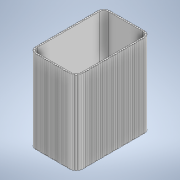
# Autodesk Inventor part: CircleContainer
Saved by Autodesk Inventor 2020 (Build 240168000, 168)
## iProperties
Created: 2024-02-26
Part Number: CircleContainer
Material: Generic
Document SubType Name: Modeling
Designer: smz3rm
Density: 1 g/cm^3
Appearance: Default
Author: smz3rm
Autodesk Inventor part; units mm, degrees
ref_plane "YZ Plane" through (0, 0, 0) normal (1, 0, 0) x (0, 1, 0)
ref_plane "XZ Plane" through (0, 0, 0) normal (0, 1, 0) x (-1, 0, 0)
ref_plane "XY Plane" through (0, 0, 0) normal (0, 0, 1) x (1, 0, 0)
sketch "Sketch3" plane through (0, 0, 0) normal (0, 1, 0) x (-1, 0, 0)
  line L0 (-31.4159, 66.9414) -> (31.4159, 66.9414)
  line L1 (41.4159, 56.9414) -> (41.4159, -56.9414)
  line L2 (31.4159, -66.9414) -> (-31.4159, -66.9414)
  line L3 (-41.4159, -56.9414) -> (-41.4159, 56.9414)
  line L4 (-41.4159, 66.9414) -> (41.4159, -66.9414) construction
  line L5 (41.4159, 66.9414) -> (-41.4159, -66.9414) construction
  arc A0 (41.4159, 56.9414) -> (31.4159, 66.9414) centre (31.4159, 56.9414) ccw
  arc A1 (-31.4159, 66.9414) -> (-41.4159, 56.9414) centre (-31.4159, 56.9414) ccw
  arc A2 (31.4159, -66.9414) -> (41.4159, -56.9414) centre (31.4159, -56.9414) ccw
  arc A3 (-41.4159, -56.9414) -> (-31.4159, -66.9414) centre (-31.4159, -56.9414) ccw
  line L6 (60.8818, 0) -> (-60.8818, 0) projected
  line L7 (0, -96.6174) -> (0, 96.6174) projected
  circle A4 centre (31.4159, 66.9414) radius 1.9635
  circle A5 centre (35.2428, 66.1802) radius 1.9635
  circle A6 centre (38.487, 64.0124) radius 1.9635
  circle A7 centre (40.6547, 60.7682) radius 1.9635
  circle A8 centre (41.4159, 56.9414) radius 1.9635
  circle A9 centre (41.4159, 53.0144) radius 1.9635
  circle A10 centre (41.4159, 49.0874) radius 1.9635
  circle A11 centre (41.4159, 45.1604) radius 1.9635
  circle A12 centre (41.4159, 41.2334) radius 1.9635
  circle A13 centre (41.4159, 37.3064) radius 1.9635
  circle A14 centre (41.4159, 33.3794) radius 1.9635
  circle A15 centre (41.4159, 29.4524) radius 1.9635
  circle A16 centre (41.4159, 25.5254) radius 1.9635
  circle A17 centre (41.4159, 21.5984) radius 1.9635
  circle A18 centre (41.4159, 17.6715) radius 1.9635
  circle A19 centre (41.4159, 13.7445) radius 1.9635
  circle A20 centre (41.4159, 9.8175) radius 1.9635
  circle A21 centre (41.4159, 5.8905) radius 1.9635
  circle A22 centre (41.4159, 1.9635) radius 1.9635
  circle A23 centre (41.4159, -1.9635) radius 1.9635
  circle A24 centre (41.4159, -5.8905) radius 1.9635
  circle A25 centre (41.4159, -9.8175) radius 1.9635
  circle A26 centre (41.4159, -13.7445) radius 1.9635
  circle A27 centre (41.4159, -17.6715) radius 1.9635
  circle A28 centre (41.4159, -21.5984) radius 1.9635
  circle A29 centre (41.4159, -25.5254) radius 1.9635
  circle A30 centre (41.4159, -29.4524) radius 1.9635
  circle A31 centre (41.4159, -33.3794) radius 1.9635
  circle A32 centre (41.4159, -37.3064) radius 1.9635
  circle A33 centre (41.4159, -41.2334) radius 1.9635
  circle A34 centre (41.4159, -45.1604) radius 1.9635
  circle A35 centre (41.4159, -49.0874) radius 1.9635
  circle A36 centre (41.4159, -53.0144) radius 1.9635
  circle A37 centre (-41.4159, 56.9414) radius 1.9635
  circle A38 centre (-41.4159, 53.0144) radius 1.9635
  circle A39 centre (-41.4159, 49.0874) radius 1.9635
  circle A40 centre (-41.4159, 45.1604) radius 1.9635
  circle A41 centre (-41.4159, 41.2334) radius 1.9635
  circle A42 centre (-41.4159, 37.3064) radius 1.9635
  circle A43 centre (-41.4159, 33.3794) radius 1.9635
  circle A44 centre (-41.4159, 29.4524) radius 1.9635
  circle A45 centre (-41.4159, 25.5254) radius 1.9635
  circle A46 centre (-41.4159, 21.5984) radius 1.9635
  circle A47 centre (-41.4159, 17.6715) radius 1.9635
  circle A48 centre (-41.4159, 13.7445) radius 1.9635
  circle A49 centre (-41.4159, 9.8175) radius 1.9635
  circle A50 centre (-41.4159, 5.8905) radius 1.9635
  circle A51 centre (-41.4159, 1.9635) radius 1.9635
  circle A52 centre (-41.4159, -1.9635) radius 1.9635
  circle A53 centre (-41.4159, -5.8905) radius 1.9635
  circle A54 centre (-41.4159, -9.8175) radius 1.9635
  circle A55 centre (-41.4159, -13.7445) radius 1.9635
  circle A56 centre (-41.4159, -17.6715) radius 1.9635
  circle A57 centre (-41.4159, -21.5984) radius 1.9635
  circle A58 centre (-41.4159, -25.5254) radius 1.9635
  circle A59 centre (-41.4159, -29.4524) radius 1.9635
  circle A60 centre (-41.4159, -33.3794) radius 1.9635
  circle A61 centre (-41.4159, -37.3064) radius 1.9635
  circle A62 centre (-41.4159, -41.2334) radius 1.9635
  circle A63 centre (-41.4159, -45.1604) radius 1.9635
  circle A64 centre (-41.4159, -49.0874) radius 1.9635
  circle A65 centre (-41.4159, -53.0144) radius 1.9635
  circle A66 centre (31.4159, -66.9414) radius 1.9635
  circle A67 centre (35.2428, -66.1802) radius 1.9635
  circle A68 centre (38.487, -64.0124) radius 1.9635
  circle A69 centre (40.6547, -60.7682) radius 1.9635
  circle A70 centre (41.4159, -56.9414) radius 1.9635
  circle A71 centre (-31.4159, 66.9414) radius 1.9635
  circle A72 centre (-35.2428, 66.1802) radius 1.9635
  circle A73 centre (-38.487, 64.0124) radius 1.9635
  circle A74 centre (-40.6547, 60.7682) radius 1.9635
  circle A75 centre (-41.4159, 56.9414) radius 1.9635
  circle A76 centre (-31.4159, -66.9414) radius 1.9635
  circle A77 centre (-35.2428, -66.1802) radius 1.9635
  circle A78 centre (-38.487, -64.0124) radius 1.9635
  circle A79 centre (-40.6547, -60.7682) radius 1.9635
  circle A80 centre (31.4159, -66.9414) radius 1.9635
  circle A81 centre (27.4889, 66.9414) radius 1.9635
  circle A82 centre (27.4889, -66.9414) radius 1.9635
  circle A83 centre (23.5619, 66.9414) radius 1.9635
  circle A84 centre (23.5619, -66.9414) radius 1.9635
  circle A85 centre (19.635, 66.9414) radius 1.9635
  circle A86 centre (19.635, -66.9414) radius 1.9635
  circle A87 centre (15.708, 66.9414) radius 1.9635
  circle A88 centre (15.708, -66.9414) radius 1.9635
  circle A89 centre (11.781, 66.9414) radius 1.9635
  circle A90 centre (11.781, -66.9414) radius 1.9635
  circle A91 centre (7.854, 66.9414) radius 1.9635
  circle A92 centre (7.854, -66.9414) radius 1.9635
  circle A93 centre (3.927, 66.9414) radius 1.9635
  circle A94 centre (3.927, -66.9414) radius 1.9635
  circle A95 centre (0, 66.9414) radius 1.9635
  circle A96 centre (0, -66.9414) radius 1.9635
  circle A97 centre (-3.927, 66.9414) radius 1.9635
  circle A98 centre (-3.927, -66.9414) radius 1.9635
  circle A99 centre (-7.854, 66.9414) radius 1.9635
  circle A100 centre (-7.854, -66.9414) radius 1.9635
  circle A101 centre (-11.781, 66.9414) radius 1.9635
  circle A102 centre (-11.781, -66.9414) radius 1.9635
  circle A103 centre (-15.708, 66.9414) radius 1.9635
  circle A104 centre (-15.708, -66.9414) radius 1.9635
  circle A105 centre (-19.635, 66.9414) radius 1.9635
  circle A106 centre (-19.635, -66.9414) radius 1.9635
  circle A107 centre (-23.5619, 66.9414) radius 1.9635
  circle A108 centre (-23.5619, -66.9414) radius 1.9635
  circle A109 centre (-27.4889, 66.9414) radius 1.9635
  circle A110 centre (-27.4889, -66.9414) radius 1.9635
  circle A111 centre (-41.4159, -56.9414) radius 1.9635
  point P0 (0, 0)
  point P1 (33.3727, 66.7785)
  point P2 (29.4524, 66.9414)
  point P3 (25.5254, 66.9414)
  point P4 (21.5984, 66.9414)
  point P5 (17.6715, 66.9414)
  point P6 (13.7445, 66.9414)
  point P7 (9.8175, 66.9414)
  point P8 (5.8905, 66.9414)
  point P9 (1.9635, 66.9414)
  point P10 (-1.9635, 66.9414)
  point P11 (-5.8905, 66.9414)
  point P12 (-9.8175, 66.9414)
  point P13 (-13.7445, 66.9414)
  point P14 (-17.6715, 66.9414)
  point P15 (-21.5984, 66.9414)
  point P16 (-25.5254, 66.9414)
  point P17 (-29.4524, 66.9414)
  point P18 (-33.3727, 66.7785)
  point P19 (-36.9882, 65.2809)
  point P20 (-39.7555, 62.5137)
  point P21 (-41.2531, 58.8981)
  point P22 (-41.4159, 54.9779)
  point P23 (-41.4159, 51.0509)
  point P24 (-41.4159, 47.1239)
  point P25 (-41.4159, 43.1969)
  point P26 (-41.4159, 39.2699)
  point P27 (-41.4159, 35.3429)
  point P28 (-41.4159, 31.4159)
  point P29 (-41.4159, 27.4889)
  point P30 (-41.4159, 23.5619)
  point P31 (-41.4159, 19.635)
  point P32 (-41.4159, 15.708)
  point P33 (-41.4159, 11.781)
  point P34 (-41.4159, 7.854)
  point P35 (-41.4159, 3.927)
  point P36 (-41.4159, 0)
  point P37 (-41.4159, -3.927)
  point P38 (-41.4159, -7.854)
  point P39 (-41.4159, -11.781)
  point P40 (-41.4159, -15.708)
  point P41 (-41.4159, -19.635)
  point P42 (-41.4159, -23.5619)
  point P43 (-41.4159, -27.4889)
  point P44 (-41.4159, -31.4159)
  point P45 (-41.4159, -35.3429)
  point P46 (-41.4159, -39.2699)
  point P47 (-41.4159, -43.1969)
  point P48 (-41.4159, -47.1239)
  point P49 (-41.4159, -51.0509)
  point P50 (-41.4159, -54.9779)
  point P51 (-41.2531, -58.8981)
  point P52 (-39.7555, -62.5137)
  point P53 (-36.9882, -65.2809)
  point P54 (-33.3727, -66.7785)
  point P55 (-29.4524, -66.9414)
  point P56 (-25.5254, -66.9414)
  point P57 (-21.5984, -66.9414)
  point P58 (-17.6715, -66.9414)
  point P59 (-13.7445, -66.9414)
  point P60 (-9.8175, -66.9414)
  point P61 (-5.8905, -66.9414)
  point P62 (-1.9635, -66.9414)
  point P63 (1.9635, -66.9414)
  point P64 (5.8905, -66.9414)
  point P65 (9.8175, -66.9414)
  point P66 (13.7445, -66.9414)
  point P67 (17.6715, -66.9414)
  point P68 (21.5984, -66.9414)
  point P69 (25.5254, -66.9414)
  point P70 (29.4524, -66.9414)
  point P71 (33.3727, -66.7785)
  point P72 (36.9882, -65.2809)
  point P73 (39.7555, -62.5137)
  point P74 (41.2531, -58.8981)
  point P75 (41.4159, -54.9779)
  point P76 (41.4159, -51.0509)
  point P77 (41.4159, -47.1239)
  point P78 (41.4159, -43.1969)
  point P79 (41.4159, -39.2699)
  point P80 (41.4159, -35.3429)
  point P81 (41.4159, -31.4159)
  point P82 (41.4159, -27.4889)
  point P83 (41.4159, -23.5619)
  point P84 (41.4159, -19.635)
  point P85 (41.4159, -15.708)
  point P86 (41.4159, -11.781)
  point P87 (41.4159, -7.854)
  point P88 (41.4159, -3.927)
  point P89 (41.4159, 0)
  point P90 (41.4159, 3.927)
  point P91 (41.4159, 7.854)
  point P92 (41.4159, 11.781)
  point P93 (41.4159, 15.708)
  point P94 (41.4159, 19.635)
  point P95 (41.4159, 23.5619)
  point P96 (41.4159, 27.4889)
  point P97 (41.4159, 31.4159)
  point P98 (41.4159, 35.3429)
  point P99 (41.4159, 39.2699)
  point P100 (41.4159, 43.1969)
  point P101 (41.4159, 47.1239)
  point P102 (41.4159, 51.0509)
  point P103 (41.4159, 54.9779)
  point P104 (41.2531, 58.8981)
  point P105 (39.7555, 62.5137)
  point P106 (36.9882, 65.2809)
  dimension "d50" = 10
  dimension "d51" = 10
  dimension "d52" = 10
  dimension "d53" = 10
  dimension "d66" = 113.8827
  dimension "d67" = 62.8319
  dimension "d68" = 3.927
  dimension "d71" = 90
  dimension "d75" = 3.927
  dimension "d78" = 82.8319
  dimension "d83" = 133.8827
  dimension "d86" = 3.927
  constraints: 112 centre point, 15 symmetric about line, 12 end point, 8 point on circle, 8 point on line, 8 tangent, 3 horizontal, 2 midpoint, 2 parallel, 2 vertical, 1 coincident, 1 perpendicular, 200 other
  measures "d50" radius of A0
  measures "d51" radius of A1
  measures "d52" radius of A2
  measures "d53" radius of A3
  measures "d66" distance of L1.end L1.start
  measures "d67" distance of L2.end L2.start
  measures "d68" diameter of A4
  measures "d75" distance of A8.centre A9.centre
  measures "d78" distance of A8.centre A37.centre
  measures "d83" distance of A4.centre A80.centre
  measures "d86" distance of A4.centre A81.centre
extrude "Extrusion3" add sketch "Sketch3" along normal blind 152.4
sketch "Sketch4" plane through (0, 152.4, 0) normal (0, 1, 0) x (1, 0, 0)
  arc A0 (-41.4159, -56.9414) -> (-31.4159, -66.9414) centre (-31.4159, -56.9414) ccw
  arc A1 (-31.4159, 66.9414) -> (-41.4159, 56.9414) centre (-31.4159, 56.9414) ccw
  arc A2 (31.4159, -66.9414) -> (41.4159, -56.9414) centre (31.4159, -56.9414) ccw
  arc A3 (41.4159, 56.9414) -> (31.4159, 66.9414) centre (31.4159, 56.9414) ccw
  line L0 (-41.4159, -56.9414) -> (-41.4159, 56.9414)
  line L1 (-31.4159, -66.9414) -> (31.4159, -66.9414)
  line L2 (41.4159, -56.9414) -> (41.4159, 56.9414)
  line L3 (-31.4159, 66.9414) -> (31.4159, 66.9414)
  line L4 (-60.8818, 0) -> (60.8818, 0) projected
  line L5 (0, 96.6174) -> (0, -96.6174) projected
  line L6 (-40.2159, 56.9414) -> (-40.2159, -56.9414)
  arc A4 (-40.2159, -56.9414) -> (-31.4159, -65.7414) centre (-31.4159, -56.9414) ccw
  line L7 (-31.4159, -65.7414) -> (31.4159, -65.7414)
  arc A5 (31.4159, -65.7414) -> (40.2159, -56.9414) centre (31.4159, -56.9414) ccw
  line L8 (40.2159, -56.9414) -> (40.2159, 56.9414)
  arc A6 (40.2159, 56.9414) -> (31.4159, 65.7414) centre (31.4159, 56.9414) ccw
  line L9 (31.4159, 65.7414) -> (-31.4159, 65.7414)
  arc A7 (-31.4159, 65.7414) -> (-40.2159, 56.9414) centre (-31.4159, 56.9414) ccw
  point P0 (0, -66.9414)
  point P1 (-41.4159, 0)
  dimension "d94" = 20
  dimension "d98" = 62.8319
  dimension "d99" = 113.8827
  dimension "d100" = 1.2
  constraints: 16 end point, 16 point on circle, 8 centre point, 8 tangent, 3 equal radius, 2 horizontal, 2 midpoint, 2 point on line, 2 vertical, 7 other
  measures "d94" diameter of A0
  measures "d98" distance of L1.start L1.end
  measures "d99" distance of L0.start L0.end
  measures "d100" distance between parallel lines of L0 L6
extrude "Extrusion4" cut sketch "Sketch4" against normal blind 149.4 contours L6 A7 L9 L5 L4 | L4 L5 L7 A4 L6 | L5 L4 L8 A5 L7 | L5 L9 A6 L8 L4
equation "\"d50\" = CornerDia"
equation "\"d51\" = CornerDia"
equation "\"d52\" = CornerDia"
equation "\"d53\" = CornerDia"
equation "\"d66\" = ActualLength"
equation "\"d67\" = ActualWidth"
equation "\"d68\" = RidgeDia"
equation "\"d75\" = RidgeDia"
equation "\"d78\" = ActualWidth + 2 * CornerDia"
equation "\"d83\" = ActualLength + 2 * CornerDia"
equation "\"d86\" = RidgeDia"
equation "\"d89\" = Height"
equation "\"d94\" = 2 * CornerDia"
equation "\"d98\" = ActualWidth"
equation "\"d99\" = ActualLength"
equation "\"d100\" = WallThickness"
equation "\"d101\" = Height - BaseThickness"
equation "\"Width\" = 75"
equation "\"Length\" = 125"
equation "\"Height\" = 152.4"
equation "\"WallThickness\" = 1.2"
equation "\"BaseThickness\" = 3"
equation "\"CornerDia\" = 10"
equation "\"ActualLength\" = 113.882734"
equation "\"ActualWidth\" = 62.831853"
equation "\"RidgeDia\" = 3.926991"
body "Solid2"
